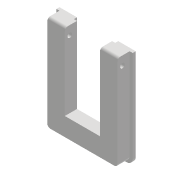
# Autodesk Inventor part: Anglerfish_coverslipclamp_top
Saved by Autodesk Inventor 2022 (Build 260153000, 153)
## iProperties
Created: 2023-04-11
Part Number: Anglerfish_coverslipclamp_top
Material: Generisch
Document SubType Name: Modeling
Designer: diederichbenedict
Density: 1 g/cm^3
Appearance: Vorgabe
Author: diederichbenedict
Autodesk Inventor part; units mm, degrees
ref_plane "YZ Plane" through (0, 0, 0) normal (1, 0, 0) x (0, 1, 0)
ref_plane "XZ Plane" through (0, 0, 0) normal (0, 1, 0) x (-1, 0, 0)
ref_plane "XY Plane" through (0, 0, 0) normal (0, 0, 1) x (1, 0, 0)
sketch "Skizze1" plane through (0, 0, 0) normal (0, 0, 1) x (1, 0, 0)
  line L0 (11.5, 38) -> (-11.5, 38)
  line L1 (-11.5, 38) -> (-11.5, -38)
  line L2 (-11.5, -38) -> (11.5, -38)
  line L3 (11.5, -38) -> (11.5, 38)
  line L4 (11.5, 38) -> (-11.5, -38) construction
  line L5 (-11.5, 38) -> (11.5, -38) construction
  line L6 (-23, -50) -> (23, -50)
  line L7 (23, -50) -> (23, -38)
  line L8 (23, -38) -> (-23, -38)
  line L9 (-23, -38) -> (-23, -50)
  line L10 (-23, -50) -> (23, -38) construction
  line L11 (23, -50) -> (-23, -38) construction
  line L12 (-23, -38) -> (-11.5, -38)
  line L13 (-11.5, -38) -> (-11.5, 12)
  line L14 (-11.5, 12) -> (-23, 12)
  line L15 (-23, 12) -> (-23, -38)
  line L16 (23, -38) -> (11.5, -38)
  line L17 (11.5, -38) -> (11.5, 12)
  line L18 (11.5, 12) -> (23, 12)
  line L19 (23, 12) -> (23, -38)
  point P0 (0, 0)
  point P1 (0, -44)
  point P2 (0, -38)
  dimension "d0" = 23
  dimension "d1" = 76
  dimension "d2" = 12
  dimension "d3" = 50
  dimension "d4" = 50
  dimension "d5" = 46
  constraints: 40 end point, 8 parallel, 6 midpoint, 4 horizontal, 4 perpendicular, 2 point on line
  measures "d0" distance of L2.end L1.end
  measures "d1" distance of L1.end L0.end
  measures "d2" distance of L7.end L6.end
  measures "d3" distance of L13.end L12.end
  measures "d4" distance of L16.end L17.end
  measures "d5" distance between parallel lines of L7 L9
extrude "Extrusion1" add sketch "Skizze1" along normal blind 10 contours L18 L19 L8 L3 | L1 L8 L15 L14 | L8 L7 L6 L9 L2
sketch "Skizze2" plane through (-11.5, -38, 0) normal (1, 0, 0) x (0, 0, -1)
  line L0 (0, 50) -> (0, -12) projected
  line L1 (0, -7.7211) -> (-0.5, -7.7211)
  line L2 (-0.5, -7.7211) -> (-2, -3.621)
  line L3 (-2, -3.621) -> (-2, 50)
  line L4 (-2, 50) -> (0, 50)
  line L5 (0, 0) -> (0, 50) projected
  point P0 (0, 38)
  point P1 (0, 5.0638)
  dimension "d8" = 0.5
  dimension "d15" = 2
  constraints: 8 end point, 2 perpendicular, 1 horizontal, 1 point on line
  measures "d8" distance of L1.start L1.end
  measures "d15" distance between parallel lines of L3 L0
extrude "Extrusion2" cut sketch "Skizze2" along normal blind 25 and the other way blind 2
sketch "Skizze3" plane through (-23, -50, 0) normal (-1, 0, 0) x (0, 0, 1)
  line L0 (0, 62) -> (0, 0) projected
  line L1 (0, 0) -> (10, 0) projected
  line L2 (10, 62) -> (10, 0) projected
  line L3 (0, 62) -> (10, 62) projected
  circle A0 centre (6.7241, 56.1881) radius 1.5
  point P0 (0, 50)
  dimension "d11" = 3
  constraints: 1 centre point
  measures "d11" diameter of A0
extrude "Extrusion3" cut sketch "Skizze3" against normal through all contours A0
fillet "Rundung1" radius 2 4 edges at (17.25, 12, 10) (-17.25, 12, 10) (-23, -50, 5) (23, -50, 5)
sketch "Skizze4" plane through (0, 0, 0) normal (0, 0, -1) x (-1, 0, 0)
  arc A0 (-23, -48) -> (-21, -50) centre (-21, -48) ccw projected
  line L0 (21, -50) -> (-21, -50) projected
  arc A1 (21, -50) -> (23, -48) centre (21, -48) ccw projected
  line L1 (23, 12) -> (23, -48) projected
  line L2 (13.5, 12) -> (23, 12) projected
  line L3 (13.5, 12) -> (13.5, -45.7211) projected
  line L4 (13.5, -45.7211) -> (-13.5, -45.7211) projected
  line L5 (-13.5, -45.7211) -> (-13.5, 12) projected
  line L6 (-23, 12) -> (-13.5, 12) projected
  line L7 (-23, -48) -> (-23, 12) projected
  line L8 (-25, 14) -> (-11.5, 14)
  line L9 (-11.5, 14) -> (-11.5, -43.7211)
  line L10 (-11.5, -43.7211) -> (11.5, -43.7211)
  line L11 (11.5, -43.7211) -> (11.5, 14)
  line L12 (11.5, 14) -> (25, 14)
  line L13 (25, 14) -> (25, -48)
  arc A2 (21, -52) -> (25, -48) centre (21, -48) ccw
  line L14 (21, -52) -> (-21, -52)
  arc A3 (-25, -48) -> (-21, -52) centre (-21, -48) ccw
  line L15 (-25, -48) -> (-25, 14)
  line L16 (-23, 12) -> (-25, 12)
  line L17 (23, 12) -> (25, 12)
  point P0 (0, 0)
  dimension "d18" = 2
  constraints: 20 end point, 4 point on circle, 2 centre point, 2 point on line, 1 horizontal, 1 perpendicular, 9 other
  measures "d18" distance between parallel lines of L7 L15
extrude "Extrusion4" add sketch "Skizze4" against normal blind 2 contours A0 L0 A1 L1 L17 L13 A2 L14 A3 L15 L16 L7
